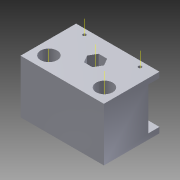
# Autodesk Inventor part: carriage
Saved by Autodesk Inventor 2013 (Build 170138000, 138)
## iProperties
Created: 2012-11-04
Part Number: carriage
Material: Generic
Document SubType Name: Modeling
Designer: Nico
Density: 1 g/cm^3
Author: Nico
Autodesk Inventor part; units mm, degrees
ref_plane "YZ Plane" through (0, 0, 0) normal (1, 0, 0) x (0, 1, 0)
ref_plane "XZ Plane" through (0, 0, 0) normal (0, 1, 0) x (-1, 0, 0)
ref_plane "XY Plane" through (0, 0, 0) normal (0, 0, 1) x (1, 0, 0)
sketch "Sketch11" plane through (0, 0, 0) normal (0, 0, 1) x (1, 0, 0)
  line L0 (3.7722, 0) -> (78.7722, 0)
  line L1 (78.7722, 0) -> (78.7722, 45)
  line L2 (78.7722, 45) -> (3.7722, 45)
  line L3 (3.7722, 45) -> (3.7722, 0)
  circle A0 centre (16.2722, 8) radius 5
  circle A1 centre (66.2722, 8) radius 5
  point P0 (0, 0)
  dimension "d63" = 75
  dimension "d65" = 45
  dimension "d66" = 10
  dimension "d67" = 10
  dimension "d68" = 50
  dimension "d69" = 12.5
  dimension "d70" = 8
  dimension "d71" = 8
  constraints: 8 end point, 2 centre point, 2 parallel, 1 horizontal, 1 perpendicular
  measures "d63" distance of L0.start L0.end
  measures "d65" distance of L2.end L0.start
  measures "d66" diameter of A1
  measures "d67" diameter of A0
  measures "d68" distance of A1.centre A0.centre
  measures "d69" distance from line of L3 A0.centre
  measures "d70" distance from line of L0 A1.centre
  measures "d71" distance from line of L0 A0.centre
extrude "Extrusion10" add sketch "Sketch11" along normal blind 5
sketch "Sketch12" plane through (0, 0, 5) normal (0, 0, 1) x (1, 0, 0)
  circle A0 centre (66.2722, 8) radius 5 projected
  circle A1 centre (16.2722, 8) radius 5 projected
  circle A2 centre (16.2722, 8) radius 7.5
  circle A3 centre (66.2722, 8) radius 7.5
  point P0 (0, 0)
  dimension "d74" = 15
  dimension "d77" = 15
  constraints: 2 centre point, 2 coincident
  measures "d74" diameter of A2
  measures "d77" diameter of A3
sketch "Sketch13" plane through (0, 0, 5) normal (0, 0, 1) x (1, 0, 0)
  line L0 (3.7722, 0) -> (78.7722, 0) projected
  line L1 (3.7722, 45) -> (3.7722, 0) projected
  line L2 (37.4644, 31.6016) -> (45.0855, 31.5984)
  line L3 (45.0855, 31.5984) -> (48.8932, 24.9968)
  line L4 (48.8932, 24.9968) -> (45.0799, 18.3984)
  line L5 (45.0799, 18.3984) -> (37.4589, 18.4016)
  line L6 (37.4589, 18.4016) -> (33.6512, 25.0032)
  line L7 (33.6512, 25.0032) -> (37.4644, 31.6016)
  point P0 (0, 0)
  point P1 (41.2722, 25)
  point P2 (41.2722, 25)
  dimension "d81" = 37.5
  dimension "d82" = 25
  dimension "d83" = 13.2
  constraints: 12 end point, 1 coincident, 13 other
  measures "d81" distance from line of L1 point (41.272, 25)
  measures "d82" distance from line of L0 point (41.272, 25)
  measures "d83" distance between parallel lines of L5 L2
sketch "Sketch14" plane through (0, 0, 5) normal (0, 0, 1) x (1, 0, 0)
  circle A0 centre (41.2722, 25) radius 5
  line L0 (3.7722, 0) -> (78.7722, 0) projected
  line L1 (3.7722, 45) -> (3.7722, 0) projected
  point P0 (0, 0)
  dimension "d87" = 10
  dimension "d89" = 25
  dimension "d90" = 37.5
  constraints: 1 centre point
  measures "d87" diameter of A0
  measures "d89" distance from line of L0 A0.centre
  measures "d90" distance from line of L1 A0.centre
extrude "Extrusion13" cut sketch "Sketch14" against normal blind 50
sketch "Sketch16" plane through (0, 0, 0) normal (0, 0, -1) x (-1, 0, 0)
  line L0 (-78.7722, 45) -> (-3.7722, 45) projected
  line L1 (-78.7722, 0) -> (-78.7722, 45) projected
  circle A0 centre (-66.2722, 40) radius 1.5
  circle A1 centre (-16.2722, 40) radius 1.5
  point P0 (0, 0)
  dimension "d99" = 3
  dimension "d101" = 3
  dimension "d102" = 5
  dimension "d103" = 5
  dimension "d104" = 50
  dimension "d105" = 12.5
  constraints: 2 centre point
  measures "d99" diameter of A0
  measures "d101" diameter of A1
  measures "d102" distance from line of A1.centre L0
  measures "d103" distance from line of L0 A0.centre
  measures "d104" distance of A0.centre A1.centre
  measures "d105" distance from line of L1 A0.centre
extrude "Extrusion15" cut sketch "Sketch16" against normal blind 100
sketch "Sketch17" plane through (3.7722, 0, 0) normal (0, -1, 0) x (1, 0, 0)
  line L0 (0, 0) -> (75, 0) projected
  line L1 (75, 0) -> (75, 5) projected
  line L2 (0, 0) -> (75, 0)
  line L3 (75, 0) -> (75, 5)
  line L4 (75, 5) -> (0, 5)
  line L5 (0, 5) -> (0, 0)
  point P0 (-3.7722, 0)
  constraints: 8 end point, 2 parallel, 1 horizontal, 1 perpendicular
extrude "Extrusion16" add sketch "Sketch17" along normal blind 5
sketch "Sketch20" plane through (0, 0, 0) normal (0, 0, -1) x (-1, 0, 0)
  circle A0 centre (-41.2722, 25) radius 5 projected
  line L0 (-45.1434, 31.4302) -> (-37.6391, 31.5677)
  line L1 (-37.6391, 31.5677) -> (-33.7679, 25.1375)
  line L2 (-33.7679, 25.1375) -> (-37.401, 18.5698)
  line L3 (-37.401, 18.5698) -> (-44.9052, 18.4323)
  line L4 (-44.9052, 18.4323) -> (-48.7765, 24.8625)
  line L5 (-48.7765, 24.8625) -> (-45.1434, 31.4302)
  point P0 (0, 0)
  dimension "d122" = 13
  constraints: 12 end point, 1 coincident, 13 other
  measures "d122" distance between parallel lines of L3 L0
extrude "Extrusion19" cut sketch "Sketch20" against normal blind 3
sketch "Sketch21" plane through (0, 0, 5) normal (0, 0, 1) x (1, 0, 0)
  circle A0 centre (41.2722, 25) radius 5 projected
  circle A1 centre (66.2722, 8) radius 5 projected
  circle A2 centre (16.2722, 8) radius 5 projected
  line L0 (78.7722, 45) -> (78.7722, -5) projected
  line L1 (78.7722, 45) -> (3.7722, 45) projected
  line L2 (3.7722, -5) -> (78.7722, -5)
  line L3 (78.7722, -5) -> (78.7722, 35)
  line L4 (78.7722, 35) -> (3.7722, 35)
  line L5 (3.7722, 35) -> (3.7722, -5)
  point P0 (0, 0)
  dimension "d125" = 10
  constraints: 8 end point, 2 parallel, 1 horizontal, 1 perpendicular, 1 point on line
  measures "d125" distance between parallel lines of L4 L1
extrude "Extrusion20" add sketch "Sketch21" along normal blind 38
extrude "Extrusion22" cut sketch "Sketch12" along normal blind 38
extrude "Extrusion23" cut sketch "Sketch13" along normal blind 38
sketch "Sketch22" plane through (0, 0, 43) normal (0, 0, 1) x (1, 0, 0)
  line L0 (45.0855, 31.5984) -> (48.8932, 24.9968) projected
  line L1 (48.8932, 24.9968) -> (45.0799, 18.3984) projected
  line L2 (45.0799, 18.3984) -> (37.4589, 18.4016) projected
  line L3 (37.4589, 18.4016) -> (33.6512, 25.0032) projected
  line L4 (33.6512, 25.0032) -> (37.4644, 31.6016) projected
  line L5 (37.4644, 31.6016) -> (45.0855, 31.5984) projected
  circle A0 centre (16.2722, 8) radius 7.5 projected
  circle A1 centre (66.2722, 8) radius 7.5 projected
  line L6 (78.7722, 35) -> (3.7722, 35) projected
  line L7 (3.7722, -5) -> (78.7722, -5)
  line L8 (78.7722, -5) -> (78.7722, 45)
  line L9 (78.7722, 45) -> (3.7722, 45)
  line L10 (3.7722, 45) -> (3.7722, -5)
  point P0 (0, 0)
  dimension "d134" = 10
  constraints: 8 end point, 2 parallel, 1 horizontal, 1 perpendicular
  measures "d134" distance between parallel lines of L9 L6
extrude "Extrusion24" add sketch "Sketch22" along normal blind 5
sketch "Sketch23" plane through (0, 0, 48) normal (0, 0, 1) x (1, 0, 0)
  line L0 (78.7722, 45) -> (3.7722, 45) projected
  line L1 (3.7722, 45) -> (3.7722, -5) projected
  circle A0 centre (16.2722, 40) radius 1.5
  circle A1 centre (66.2722, 40) radius 1.5
  point P0 (0, 0)
  dimension "d137" = 3
  dimension "d139" = 3
  dimension "d140" = 50
  dimension "d141" = 12.5
  dimension "d142" = 5
  dimension "d143" = 5
  constraints: 2 centre point
  measures "d137" diameter of A0
  measures "d139" diameter of A1
  measures "d140" distance of A1.centre A0.centre
  measures "d141" distance from line of A0.centre L1
  measures "d142" distance from line of A0.centre L0
  measures "d143" distance from line of A1.centre L0
extrude "Extrusion25" cut sketch "Sketch23" against normal blind 5
body "Solid2"
